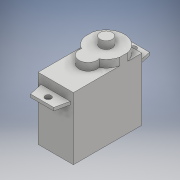
# Autodesk Inventor part: RB-001-Servo
Saved by Autodesk Inventor 2018.3 (Build 223284000, 284)
## iProperties
Created: 2019-02-13
Part Number: RB-001-Servo
Material: 一般
Document SubType Name: Modeling
Designer: shun2
Density: 1 g/cm^3
Appearance: 既定
Author: shun2
Autodesk Inventor part; units mm, degrees
ref_plane "YZ Plane" through (0, 0, 0) normal (1, 0, 0) x (0, 1, 0)
ref_plane "XZ Plane" through (0, 0, 0) normal (0, 1, 0) x (-1, 0, 0)
ref_plane "XY Plane" through (0, 0, 0) normal (0, 0, 1) x (1, 0, 0)
sketch "スケッチ1" plane through (0, 0, 0) normal (0, 0, 1) x (1, 0, 0)
  line L0 (0, 0) -> (11.7, 0)
  line L1 (11.7, 0) -> (11.7, 22.7)
  line L2 (11.7, 22.7) -> (0, 22.7)
  line L3 (0, 22.7) -> (0, 0)
  dimension "d0" = 11.7
  dimension "d1" = 22.7
  constraints: 8 end point, 2 parallel, 1 horizontal, 1 perpendicular
  measures "d0" distance of L2.end L1.end
  measures "d1" distance of L1.end L0.end
extrude "押し出し1" add sketch "スケッチ1" along normal blind 20.7
sketch "スケッチ2" plane through (0, 0, 20.7) normal (0, 0, 1) x (1, 0, 0)
  line L0 (11.7, 22.7) -> (0, 22.7) projected
  arc A0 (2.9453, 11.45) -> (8.7547, 11.45) centre (5.85, 10.7) ccw
  line L1 (0, 22.7) -> (0, 0) projected
  line L2 (11.7, 0) -> (11.7, 22.7) projected
  arc A1 (0, 15.3668) -> (2.9453, 11.45) centre (5.85, 16.7) ccw
  arc A2 (8.7547, 11.45) -> (11.7, 15.3668) centre (5.85, 16.7) ccw
  arc A3 (11.7, 18.0332) -> (0, 18.0332) centre (5.85, 16.7) ccw
  dimension "d5" = 6
  dimension "d6" = 6
  constraints: 8 point on circle, 4 centre point, 4 point on line
  measures "d5" distance from line of L0 A1.centre
  measures "d6" diameter of A0
extrude "押し出し2" add sketch "スケッチ2" along normal blind 2.5 contours A3 L2 A2 A0 A1 L1
sketch "スケッチ3" plane through (0, 0, 23.2) normal (0, 0, 1) x (1, 0, 0)
  arc A0 (11.7, 18.0332) -> (0, 18.0332) centre (5.85, 16.7) ccw projected
  circle A1 centre (5.85, 16.7) radius 2
  point P0 (0, 0)
  dimension "d9" = 4
  constraints: 1 centre point, 1 coincident
  measures "d9" diameter of A1
extrude "押し出し3" add sketch "スケッチ3" along normal blind 2.5
sketch "スケッチ4" plane through (0, 0, 0) normal (0, -1, 0) x (1, 0, 0)
  line L0 (11.7, 0) -> (11.7, 20.7) projected
  line L1 (0, 17.7) -> (11.7, 17.7)
  line L2 (11.7, 17.7) -> (11.7, 16.7)
  line L3 (11.7, 16.7) -> (0, 16.7)
  line L4 (0, 16.7) -> (0, 17.7)
  point P0 (0, 0)
  dimension "d12" = 1
  constraints: 8 end point, 2 parallel, 1 horizontal, 1 perpendicular, 1 point on line
  measures "d12" distance of L1.end L2.end
extrude "押し出し4" add sketch "スケッチ4" along normal blind 4.5
sketch "スケッチ5" plane through (0, 22.7, 0) normal (0, 1, 0) x (1, 0, 0)
  line L0 (11.7, -17.7) -> (11.7, -20.7) projected
  line L1 (11.7, -17.7) -> (0, -17.7)
  line L2 (0, -17.7) -> (0, -16.7)
  line L3 (0, -16.7) -> (11.7, -16.7)
  line L4 (11.7, -16.7) -> (11.7, -17.7)
  point P0 (0, 0)
  dimension "d15" = 1
  constraints: 8 end point, 2 parallel, 1 horizontal, 1 perpendicular
  measures "d15" distance of L1.end L2.end
extrude "押し出し5" add sketch "スケッチ5" along normal blind 4.5
sketch "スケッチ6" plane through (0, 0, 17.7) normal (0, 0, 1) x (1, 0, 0)
  line L0 (0, -4.5) -> (11.7, -4.5) projected
  line L1 (2, -4.5) -> (1, 0)
  line L2 (0, 0) -> (11.7, 0) projected
  line L3 (10.7, 0) -> (9.7, -4.5)
  line L4 (0, 27.2) -> (11.7, 27.2) projected
  line L5 (5.85, 22.7) -> (0, 22.7) projected
  line L6 (1.5, 22.7) -> (2, 27.2)
  line L7 (11.7, 22.7) -> (0, 22.7) projected
  line L8 (10.7, 22.7) -> (9.7, 27.2)
  circle A0 centre (5.85, 25.7) radius 1
  circle A1 centre (5.85, -2.5) radius 1
  line L9 (11.7, -4.5) -> (11.7, 0)
  line L10 (0, 0) -> (0, -4.5)
  line L11 (0, 22.7) -> (0, 27.2)
  line L12 (11.7, 27.2) -> (11.7, 22.7)
  line L13 (0, -4.5) -> (0, 0)
  line L14 (11.7, 0) -> (11.7, -4.5)
  line L15 (0, 22.7) -> (0, 27.2)
  line L16 (11.7, 27.2) -> (11.7, 22.7)
  line L17 (11.7, -4.5) -> (9.7, -4.5)
  line L18 (2, -4.5) -> (0, -4.5)
  line L19 (0, 0) -> (1, 0)
  line L20 (10.7, 0) -> (11.7, 0)
  line L21 (11.7, 22.7) -> (10.7, 22.7)
  line L22 (1.5, 22.7) -> (0, 22.7)
  line L23 (0, 27.2) -> (2, 27.2)
  line L24 (9.7, 27.2) -> (11.7, 27.2)
  dimension "d18" = 2
  dimension "d19" = 2
  constraints: 40 end point, 12 parallel, 4 horizontal, 4 perpendicular, 4 point on line, 2 centre point, 1 collinear, 1 vertical
  measures "d18" diameter of A0
  measures "d19" diameter of A1
extrude "押し出し6" cut sketch "スケッチ6" against normal blind 4.5 contours L10 L2 L1 L0 | L3 L2 L9 L0 | L4 L6 L5 L11 | L4 L12 L7 L8 | A0 | A1
sketch "スケッチ7" plane through (0, 22.7, 0) normal (0, 1, 0) x (1, 0, 0)
  line L0 (3.1, -2.5) -> (8.6, -2.5)
  line L1 (8.6, -2.5) -> (8.6, -5.5)
  line L2 (8.6, -5.5) -> (3.1, -5.5)
  line L3 (3.1, -5.5) -> (3.1, -2.5)
  line L4 (0, 0) -> (0, -20.7) projected
  dimension "d22" = 5.5
  dimension "d23" = 3
  constraints: 8 end point, 2 parallel, 1 horizontal, 1 perpendicular
  measures "d22" distance of L1.end L2.end
  measures "d23" distance of L0.end L1.end
extrude "押し出し7" add sketch "スケッチ7" along normal blind 3
